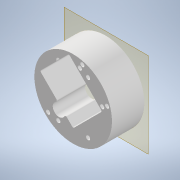
# Autodesk Inventor part: Matchboxscope_focusingblock_v0
Saved by Autodesk Inventor 2022 (Build 260153000, 153)
## iProperties
Created: 2022-05-17
Part Number: Matchboxscope_focusingblock_v0
Material: Generisch
Document SubType Name: Modeling
Designer: diederichbenedict
Density: 1 g/cm^3
Appearance: Vorgabe
Author: diederichbenedict
Autodesk Inventor part; units mm, degrees
ref_plane "YZ Plane" through (0, 0, 0) normal (1, 0, 0) x (0, 1, 0)
ref_plane "XZ Plane" through (0, 0, 0) normal (0, 1, 0) x (-1, 0, 0)
ref_plane "Arbeitsebene1" through (0, 0, 0) normal (0, 0, 1) x (1, 0, 0)
sketch "Skizze1" plane through (0, 0, 0) normal (0, 0, 1) x (1, 0, 0)
  circle A0 centre (-9.9998, 17.4978) radius 1.3999 projected
  circle A1 centre (10.0001, 17.4979) radius 1.4 projected
  circle A2 centre (10.0001, -17.5021) radius 1.4 projected
  circle A3 centre (-9.9999, -17.5021) radius 1.4001 projected
  circle A4 centre (4.4725, 20.2023) radius 1.4 projected
  circle A5 centre (19.4212, 5.2535) radius 1.4 projected
  circle A6 centre (0.0001, -0.0022) radius 6.7754 projected
  arc A7 (-25.1198, 6.6998) -> (-24.1417, 5.4917) centre (-24.1417, 6.4917) ccw projected
  line L0 (-24.1417, 5.4917) -> (-17.7002, 5.4917) projected
  arc A8 (-15.7002, 3.4917) -> (-17.7002, 5.4917) centre (-17.7002, 3.4917) ccw projected
  line L1 (-15.7002, 3.4917) -> (-15.7002, -4.496) projected
  arc A9 (-17.7002, -6.496) -> (-15.7002, -4.496) centre (-17.7002, -4.496) ccw projected
  line L2 (-17.7002, -6.496) -> (-23.8502, -6.496) projected
  arc A10 (-23.8502, -6.496) -> (-24.8235, -7.7254) centre (-23.8502, -7.496) ccw projected
  arc A11 (-24.8235, -7.7254) -> (-25.1198, 6.6998) centre (0, 0) ccw projected
  circle A12 centre (-9.4998, -11.0022) radius 2.6601 projected
  circle A13 centre (-16.8291, -16.0481) radius 1.4 projected
  circle A14 centre (6.1284, 23.0202) radius 1.4 projected
  circle A15 centre (22.7119, 7.1872) radius 1.4 projected
  arc A16 (-25.1198, 6.6998) -> (-24.6232, -8.3421) centre (0, 0) ccw
  circle A17 centre (-9.4998, -11.0022) radius 4.196
  point P0 (0, 0)
  constraints: 3 point on circle, 2 centre point, 2 concentric, 1 coincident
ref_plane "Arbeitsebene2" through (-21.5666, -16.2656, 21.7) normal (0, 0, 1) x (0.7071, -0.7071, 0)
extrude "Extrusion1" add sketch "Skizze1" along normal up to surface (21.7 mm away) contours A11 A10 L2 A9 L1 A8 L0 A7 | A7 L0 A8 L1 A9 L2 A10 A16
sketch "Skizze2" plane through (-24.1417, 5.4917, 21.7) normal (0, 0, 1) x (1, 0, 0)
  arc A0 (30.5656, -11.7979) -> (31.153, -11.2105) centre (30.5058, -11.1507) ccw projected
  line L0 (30.5656, -11.7979) -> (24.8489, -17.5146) projected
  line L1 (24.8489, -17.5146) -> (19.6708, -12.3365) projected
  arc A1 (17.2991, -9.9648) -> (19.6708, -12.3365) centre (18.1314, -11.5042) ccw projected
  line L2 (17.2991, -9.9648) -> (12.8281, -5.4938) projected
  line L3 (12.8281, -5.4938) -> (15.7017, -2.6202) projected
  arc A2 (17.7327, -0.5892) -> (15.7017, -2.6202) centre (16.0101, -0.8976) ccw projected
  line L4 (17.7327, -0.5892) -> (24.1418, 5.8199) projected
  line L5 (24.1418, 5.8199) -> (28.7374, 1.2243) projected
  arc A3 (30.8599, -0.8982) -> (28.7374, 1.2243) centre (30.435, 0.7994) ccw projected
  line L6 (30.8599, -0.8982) -> (36.1626, -6.2009) projected
  line L7 (36.1626, -6.2009) -> (34.5533, -7.8102) projected
  arc A4 (32.1151, -10.2485) -> (34.5533, -7.8102) centre (33.5463, -9.2415) ccw projected
  line L8 (32.1151, -10.2485) -> (31.153, -11.2105) projected
  circle A5 centre (12.8281, -4.0796) radius 0.65 projected
  line L9 (21.2427, 4.9006) -> (17.8485, 8.2948) projected
  line L10 (17.8485, 8.2948) -> (14.4544, 11.6889) projected
  line L11 (14.4544, 11.6889) -> (2.575, -0.1905) projected
  line L12 (2.575, -0.1905) -> (24.1418, -21.7573) projected
  line L13 (24.1418, -21.7573) -> (42.8094, -3.0897) projected
  line L14 (42.8094, -3.0897) -> (28.0309, 11.6889) projected
  line L15 (28.0309, 11.6889) -> (24.6368, 8.2948) projected
  line L16 (24.6368, 8.2948) -> (21.2427, 4.9006) projected
  circle A6 centre (21.2427, 11.6889) radius 4.8 projected
  line L17 (42.8094, -3.0897) -> (24.1418, -21.7573)
  line L18 (24.1418, -21.7573) -> (2.575, -0.1905)
  line L19 (2.575, -0.1905) -> (21.2427, 18.4771)
  line L20 (21.2427, 18.4771) -> (42.8094, -3.0897)
  line L21 (21.2427, 19.1842) -> (1.8679, -0.1905)
  line L22 (1.8679, -0.1905) -> (24.1418, -22.4644)
  line L23 (24.1418, -22.4644) -> (43.5165, -3.0897)
  line L24 (43.5165, -3.0897) -> (21.2427, 19.1842)
  point P0 (24.1417, -5.4917)
  dimension "d2" = 0.5
  constraints: 16 end point, 5 equal length, 2 perpendicular, 3 other
  measures "d2" distance between parallel lines of L19 L21
extrude "Extrusion2" cut sketch "Skizze2" against normal through all contours L0 L1 A1 L2 L3 A2 L4 L5 A3 L6 L7 A4 L8 A0 | A5 | L16 L15 L14 L13 L12 L11 L10 L9 | L9 A6 L16 | A6 | L10 L19 A6 | A6 L20 L15 | L19 L20 A6 | L24 L23 L22 L21
fillet "Rundung1" radius 1 8 edges at (-2.899, 24.6759, 10.85) (19.3748, 2.402, 10.85) (0.0001, -16.9727, 10.85) (-22.2737, 5.3011, 10.85) (-10.1203, -6.8523, 10.85) (-5.3499, -11.6226, 10.85) (-11.0276, 16.5473, 10.85) (-9.0493, 18.5256, 10.85)
